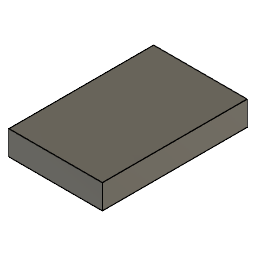
InkTime_case_assembly (Autodesk Fusion 360 archive; units mm, degrees)
design "LP502030 Li-Po battery"
part number: 2026-03-25-17-36-51-763
Autodesk Fusion 360 part; units mm, degrees
sketch "Esquisse1" plane through (0, 0, 0) normal (0, 0, 1) x (1, 0, 0)
  line L0 (0, 0) -> (21, 0)
  line L1 (21, 0) -> (21, 32.5)
  line L2 (21, 32.5) -> (0, 32.5)
  line L3 (0, 32.5) -> (0, 0)
  dimension "d1" = 21
  dimension "d2" = 32.5
  constraint horizontal L0
  constraint vertical L1
  constraint horizontal L2
  constraint vertical L3
  constraint coincident L0.start L3.end
  measures "d1" distance of L0.start L0.end
  measures "d2" distance of L0.start L2.end
extrude "Extrusion1" add sketch "Esquisse1" along normal blind 5.5

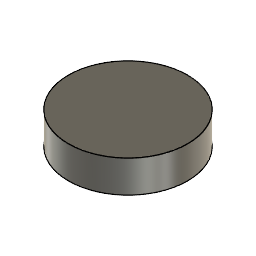
design "FIT0774 - Vibration Motor(shaker)"
part number: 2026-03-25-17-48-16-187
Autodesk Fusion 360 part; units mm, degrees
sketch "Esquisse1" plane through (0, 0, 0) normal (0, 0, 1) x (1, 0, 0)
  circle A0 centre (0, 0) radius 5
  dimension "d1" = 10
  constraint coincident A0.centre origin
  measures "d1" diameter of A0
extrude "Extrusion1" add sketch "Esquisse1" along normal blind 2.7

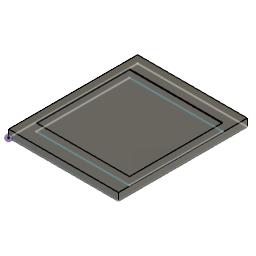
design "E-Paper Display"
part number: 2026-03-25-17-51-57-383
Autodesk Fusion 360 part; units mm, degrees
sketch "Esquisse1" plane through (0, 0, 0) normal (0, 0, 1) x (1, 0, 0)
  line L0 (0, 0) -> (31.8, 0)
  line L1 (31.8, 0) -> (31.8, 37.32)
  line L2 (31.8, 37.32) -> (0, 37.32)
  line L3 (0, 37.32) -> (0, 0)
  line L4 (2.4, 32.5871) -> (29.4, 32.5871)
  line L5 (29.4, 32.5871) -> (29.4, 5.5871)
  line L6 (29.4, 5.5871) -> (2.4, 5.5871)
  line L7 (2.4, 5.5871) -> (2.4, 32.5871)
  dimension "d1" = 37.32
  dimension "d2" = 31.8
  dimension "d3" = 2.4
  dimension "d4" = 27
  dimension "d5" = 27
  constraint horizontal L0
  constraint vertical L1
  constraint horizontal L2
  constraint vertical L3
  constraint coincident L0.start L3.end
  constraint horizontal L4
  constraint vertical L5
  constraint horizontal L6
  constraint vertical L7
  measures "d1" distance of L0.start L2.end
  measures "d2" distance of L0.start L0.end
  measures "d3" distance of L1 L5
  measures "d4" distance of L4.start L4.end
  measures "d5" distance of L4.end L5.end
extrude "Extrusion1" add sketch "Esquisse1" along normal blind 2 contours L4 L5 L6 L7
sketch "Esquisse2" plane through (0, 0, 0) normal (0, 0, 1) x (1, 0, 0)
extrude "Extrusion2" add sketch "Esquisse1" along normal blind 2.2
